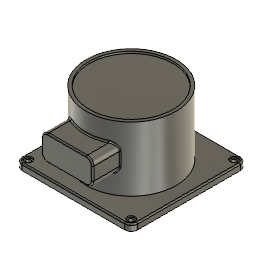
Base of robotic arm (Autodesk Fusion 360 design; units mm, degrees)
part number: 2025-12-13-21-49-26-084
Autodesk Fusion 360 part; units mm, degrees
sketch "Sketch1" plane through (0, 0, 0) normal (0, 0, 1) x (1, 0, 0)
  line L0 (-90, 90) -> (90, 90)
  line L1 (90, 90) -> (90, -90)
  line L2 (90, -90) -> (-90, -90)
  line L3 (-90, -90) -> (-90, 90)
  line L4 (-90, 90) -> (90, -90) construction
  line L5 (90, 90) -> (-90, -90) construction
  dimension "d1" = 180
  dimension "d2" = 180
  constraint horizontal L0
  constraint perpendicular L0 L1
  constraint parallel L0 L2
  constraint parallel L1 L3
  constraint coincident L4 origin
  constraint coincident L5 origin
  measures "d1" distance of L0.end L1.end
  measures "d2" distance of L0.start L0.end
extrude "Extrude1" add sketch "Sketch1" along normal blind 10
sketch "Sketch2" plane through (0, 0, 10) normal (0, 0, 1) x (-1, 0, 0)
  line L0 (90, 90) -> (-90, 90)
  line L1 (-90, 90) -> (-90, -90)
  line L2 (-90, -90) -> (90, -90)
  line L3 (90, -90) -> (90, 90)
  circle A0 centre (0, 0) radius 70
  dimension "d5" = 140
  constraint coincident A0.centre origin
  measures "d5" diameter of A0
extrude "Extrude2" add sketch "Sketch2" along normal blind 100 contours A0
sketch "Sketch3" plane through (0, 0, 0) normal (0, 1, 0) x (1, 0, 0)
  line L0 (-40, -80) -> (40, -80)
  line L1 (40, -80) -> (40, -40)
  line L2 (40, -40) -> (-40, -40)
  line L3 (-40, -40) -> (-40, -80)
  line L4 (-40, -80) -> (40, -40) construction
  line L5 (40, -80) -> (-40, -40) construction
  point P0 (0, -60)
  dimension "d13" = 40
  dimension "d14" = 80
  dimension "d16" = 60
  constraint horizontal L0
  constraint perpendicular L0 L1
  constraint parallel L0 L2
  constraint parallel L1 L3
  constraint coincident L4 P0
  constraint coincident L5 P0
  measures "d13" distance of L0.start L2.end
  measures "d14" distance of L0.start L0.end
  measures "d16" distance of origin P0
extrude "Extrude3" add sketch "Sketch3" against normal blind 100
sketch "Sketch4" plane through (0, 0, 110) normal (0, 0, 1) x (-1, 0, 0)
  circle A0 centre (0, 0) radius 70
  circle A1 centre (0, 0) radius 65
  dimension "d10" = -5
extrude "Extrude4" cut sketch "Sketch4" against normal blind 10 contours A1
extrude "Extrude5" add 1 faces at (2.3225, -16.9397, 100) along direction (0, 0, 1) blind 7
sketch "Sketch5" plane through (0, 0, 10) normal (0, 0, 1) x (-1, 0, 0)
  circle A0 centre (0, 0) radius 70
  line L0 (90, 90) -> (-90, 90)
  line L1 (-90, 90) -> (-90, -90)
  line L2 (-90, -90) -> (90, -90)
  line L3 (90, -90) -> (90, 90)
  point P0 (80, -80)
  point P1 (-80, -80)
  point P2 (-80, 80)
  point P3 (80, 80)
  point P4 (116.0582, 65.2033)
  dimension "d19" = 10
  dimension "d20" = 10
  dimension "d21" = 10
  dimension "d22" = 10
  dimension "d23" = 10
  dimension "d24" = 10
  dimension "d25" = 10
  dimension "d26" = 10
  constraint horizontal P0 P1
  constraint vertical P1 P2
  constraint horizontal P2 P3
  measures "d19" vertical distance of L0.start P3
  measures "d20" horizontal distance of L0.start P3
  measures "d21" distance of L2 P1
  measures "d22" distance of L1 P1
  measures "d23" vertical distance of L0.start P2
  measures "d24" distance of L1 P2
  measures "d25" distance of L2 P0
  measures "d26" distance of L3 P0
hole "Hole1" at (-80, -80, 10) at (80, -80, 10) at (80, 80, 10) at (-80, 80, 10) direction (0, 0, -1) diameter 7 depth 15 tip angle 118 counterbore diameter 12 counterbore depth 2
fillet "Fillet1" radius 10 8 edges at (-90, -90, 5) (90, -90, 5) (90, 90, 5) (-90, 90, 5) (40, -78.7228, 80) (40, -78.7228, 40) (-40, -78.7228, 80) (-40, -78.7228, 40)
fillet "Fillet2" radius 2 24 edges at (87.0711, -87.0711, 10) (90, 0, 10) (87.0711, 87.0711, 10) (0, 90, 10) (-87.0711, 87.0711, 10) (-90, 0, 10) (-87.0711, -87.0711, 10) (0, -90, 10) (-37.0711, -100, 77.0711) (-40, -100, 60) (-37.0711, -100, 42.9289) (0, -100, 40) (37.0711, -100, 42.9289) (40, -100, 60) (37.0711, -100, 77.0711) (0, -100, 80) (36.9012, -59.4835, 77.2363) (40, -57.4456, 60) (36.9012, -59.4835, 42.7637) (0, -70, 40) (-36.9012, -59.4835, 42.7637) (-40, -57.4456, 60) (-36.9012, -59.4835, 77.2363) (0, -70, 80)
